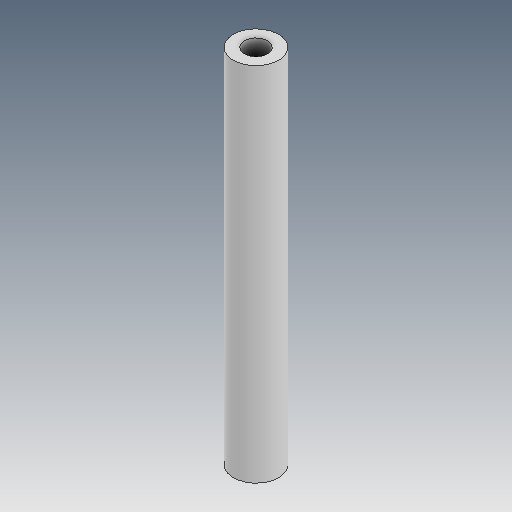
# Autodesk Inventor part: spacer
Saved by Autodesk Inventor 2025.4 (Build 294407020, 407B)
## iProperties
Created: 2026-09-08
Part Number: spacer
Material: Generic
Document SubType Name: Modeling
Designer: Aiden
Density: 1 g/cm^3
Appearance: Default
Author: Aiden
Autodesk Inventor part; units mm, degrees
ref_plane "YZ Plane" through (0, 0, 0) normal (1, 0, 0) x (0, 1, 0)
ref_plane "XZ Plane" through (0, 0, 0) normal (0, 1, 0) x (-1, 0, 0)
ref_plane "XY Plane" through (0, 0, 0) normal (0, 0, 1) x (1, 0, 0)
sketch "Sketch2" plane through (0, 0, 0) normal (0, 1, 0) x (-1, 0, 0)
  circle A0 centre (0, 0) radius 5
  circle A1 centre (0, 0) radius 2.55
  dimension "d4" = 10
  dimension "d5" = 5.1
  constraints: 2 centre point, 2 coincident
  measures "d4" diameter of A0
  measures "d5" diameter of A1
extrude "Extrusion2" add sketch "Sketch2" along normal blind 80
body "Solid2"
